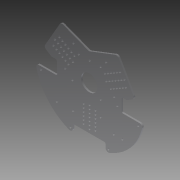
# Autodesk Inventor part: Motor Mount Plate
Saved by Autodesk Inventor 2015 (Build 190159000, 159)
## iProperties
Created: 2016-02-17
Part Number: Motor Mount Plate
Material: Polycarbonate, Clear
Document SubType Name: Modeling
Designer: 23902
Density: 1.2 g/cm^3
Appearance: Polycarbonate - Clear
Mass: 81.7977 g
Surface Area: 498.85 cm^2
Volume: 68.1648 cm^3
Author: 23902
Autodesk Inventor part; units mm, degrees
ref_plane "YZ Plane" through (0, 0, 0) normal (1, 0, 0) x (0, 1, 0)
ref_plane "XZ Plane" through (0, 0, 0) normal (0, 1, 0) x (-1, 0, 0)
ref_plane "XY Plane" through (0, 0, 0) normal (0, 0, 1) x (1, 0, 0)
sketch "Sketch1" plane through (0, 0, 0) normal (0, 1, 0) x (-1, 0, 0)
  circle A0 centre (63.7847, 36.7947) radius 1.65
  circle A1 centre (58.2854, 33.6197) radius 1.65
  circle A2 centre (52.7862, 30.4447) radius 1.65
  circle A3 centre (47.2869, 27.2697) radius 1.65
  circle A4 centre (41.7877, 24.0947) radius 1.65
  circle A5 centre (36.2884, 20.9197) radius 1.65
  circle A6 centre (30.7891, 17.7447) radius 1.65
  circle A7 centre (55.675, 44.6411) radius 1.65
  circle A8 centre (50.1758, 41.4661) radius 1.65
  circle A9 centre (44.6765, 38.2911) radius 1.65
  circle A10 centre (39.1772, 35.1161) radius 1.65
  circle A11 centre (33.678, 31.9411) radius 1.65
  circle A12 centre (28.1787, 28.7661) radius 1.65
  circle A13 centre (66.525, 25.8483) radius 1.65
  circle A14 centre (61.0258, 22.6733) radius 1.65
  circle A15 centre (55.5265, 19.4983) radius 1.65
  circle A16 centre (50.0272, 16.3233) radius 1.65
  circle A17 centre (44.528, 13.1483) radius 1.65
  circle A18 centre (39.0287, 9.9733) radius 1.65
  circle A19 centre (-63.6942, 36.7947) radius 1.65
  circle A20 centre (-58.195, 33.6197) radius 1.65
  circle A21 centre (-52.6957, 30.4447) radius 1.65
  circle A22 centre (-47.1965, 27.2697) radius 1.65
  circle A23 centre (-41.6972, 24.0947) radius 1.65
  circle A24 centre (-36.1979, 20.9197) radius 1.65
  circle A25 centre (-30.6987, 17.7447) radius 1.65
  circle A26 centre (-55.5846, 44.6411) radius 1.65
  circle A27 centre (-50.0853, 41.4661) radius 1.65
  circle A28 centre (-44.586, 38.2911) radius 1.65
  circle A29 centre (-39.0868, 35.1161) radius 1.65
  circle A30 centre (-33.5875, 31.9411) radius 1.65
  circle A31 centre (-28.0883, 28.7661) radius 1.65
  circle A32 centre (-66.4346, 25.8483) radius 1.65
  circle A33 centre (-60.9353, 22.6733) radius 1.65
  circle A34 centre (-55.436, 19.4983) radius 1.65
  circle A35 centre (-49.9368, 16.3233) radius 1.65
  circle A36 centre (-44.4375, 13.1483) radius 1.65
  circle A37 centre (-38.9383, 9.9733) radius 1.65
  circle A38 centre (0.0452, -73.6053) radius 1.65
  circle A39 centre (0.0452, -67.2553) radius 1.65
  circle A40 centre (0.0452, -60.9053) radius 1.65
  circle A41 centre (0.0452, -54.5553) radius 1.65
  circle A42 centre (0.0452, -48.2053) radius 1.65
  circle A43 centre (0.0452, -41.8553) radius 1.65
  circle A44 centre (0.0452, -35.5053) radius 1.65
  circle A45 centre (10.8952, -70.5053) radius 1.65
  circle A46 centre (10.8952, -64.1553) radius 1.65
  circle A47 centre (10.8952, -57.8053) radius 1.65
  circle A48 centre (10.8952, -51.4553) radius 1.65
  circle A49 centre (10.8952, -45.1053) radius 1.65
  circle A50 centre (10.8952, -38.7553) radius 1.65
  circle A51 centre (-10.8048, -70.5053) radius 1.65
  circle A52 centre (-10.8048, -64.1553) radius 1.65
  circle A53 centre (-10.8048, -57.8053) radius 1.65
  circle A54 centre (-10.8048, -51.4553) radius 1.65
  circle A55 centre (-10.8048, -45.1053) radius 1.65
  circle A56 centre (-10.8048, -38.7553) radius 1.65
  circle A57 centre (-29.9548, 47.4947) radius 1.6
  circle A58 centre (30.0452, 47.4947) radius 1.6
  circle A59 centre (35.0452, -88.3229) radius 1.6
  circle A60 centre (-34.9548, -88.3229) radius 1.6
  circle A61 centre (-89.3029, -23.9461) radius 1.6
  circle A62 centre (89.3934, -23.9461) radius 1.6
  circle A63 centre (-20.3391, -44.6576) radius 1.6079
  circle A64 centre (30.4218, -59.8922) radius 1.6079
  circle A65 centre (-44.4606, -59.8922) radius 1.6079
  circle A66 centre (-50.7872, -11.6704) radius 1.6079
  circle A67 centre (-20.3391, -16.7486) radius 1.6079
  circle A68 centre (31.6913, -11.6704) radius 1.6079
  circle A69 centre (0.0452, -0.0053) radius 15
  circle A70 centre (-19.9548, 34.9947) radius 1.6
  circle A71 centre (20.0452, 34.9947) radius 1.6
  circle A72 centre (60.1493, -60.1094) radius 1.6
  circle A73 centre (-60.0588, -60.1094) radius 1.6
  circle A74 centre (0.0452, 34.9947) radius 1.6
  circle A75 centre (45.0452, -0.0053) radius 1.6
  circle A76 centre (-44.9548, -0.0053) radius 1.6
  line L0 (0.0452, -80.0053) -> (-15.8048, -80.0053)
  line L1 (69.3273, 39.9947) -> (54.1439, 66.293)
  line L2 (-69.2368, 39.9947) -> (-54.0534, 66.293)
  line L3 (1.8413, 50.686) -> (48.0177, 68.4593)
  line L4 (-1.7508, 50.686) -> (-47.9273, 68.4593)
  arc A77 (-47.9273, 68.4593) -> (-54.0534, 66.293) centre (-49.7233, 63.793) ccw
  arc A78 (54.1439, 66.293) -> (48.0177, 68.4593) centre (49.8138, 63.793) ccw
  arc A79 (-1.7508, 50.686) -> (1.8413, 50.686) centre (0.0452, 55.3523) ccw
  line L5 (0.0452, -80.0053) -> (-27.9548, -80.0053)
  line L6 (-29.9548, -82.0053) -> (-29.9548, -88.3229)
  arc A80 (-44.5963, -89.4879) -> (-36.7969, -92.9712) centre (0.0452, -0.0053) ccw
  arc A81 (-36.7969, -92.9712) -> (-29.9548, -88.3229) centre (-34.9548, -88.3229) ccw
  arc A82 (-27.9548, -80.0053) -> (-29.9548, -82.0053) centre (-27.9548, -82.0053) ccw
  line L7 (0.0452, -80.0053) -> (15.8952, -80.0053)
  line L8 (0.0452, -80.0053) -> (28.0452, -80.0053)
  arc A83 (30.0452, -82.0053) -> (28.0452, -80.0053) centre (28.0452, -82.0053) ccw
  line L9 (30.0452, -82.0053) -> (30.0452, -88.3229)
  arc A84 (36.8873, -92.9712) -> (44.6868, -89.4879) centre (0.0452, -0.0053) ccw
  arc A85 (30.0452, -88.3229) -> (36.8873, -92.9712) centre (35.0452, -88.3229) ccw
  line L10 (-69.2368, 39.9947) -> (-80.8207, 19.9307)
  line L11 (-89.3029, -17.9461) -> (-92.1433, -17.9461)
  line L12 (-89.3029, -17.9461) -> (-71.3029, -17.9461)
  line L13 (-69.7888, 7.357) -> (-79.137, 13.1885)
  arc A86 (-96.9953, -24.1535) -> (-44.5963, -89.4879) centre (0.0452, -0.0053) ccw
  arc A87 (-92.1433, -17.9461) -> (-96.9953, -24.1535) centre (-92.1433, -22.9461) ccw
  arc A88 (-80.8207, 19.9307) -> (-79.137, 13.1885) centre (-76.4906, 17.4307) ccw
  line L14 (69.3273, 39.9947) -> (80.9112, 19.9307)
  arc A89 (79.2274, 13.1885) -> (80.9112, 19.9307) centre (76.5811, 17.4307) ccw
  arc A90 (44.6868, -89.4879) -> (97.0858, -24.1535) centre (0.0452, -0.0053) ccw
  arc A91 (97.0858, -24.1535) -> (92.2337, -17.9461) centre (92.2337, -22.9461) ccw
  line L15 (-71.3029, -17.9461) -> (-69.3029, -17.9461)
  line L16 (-69.3029, -17.9461) -> (-61.3029, -17.9461)
  line L17 (-59.3029, -15.9461) -> (-59.3029, 5.0539)
  line L18 (-61.3029, 7.0539) -> (-68.7302, 7.0539)
  arc A92 (-61.3029, -17.9461) -> (-59.3029, -15.9461) centre (-61.3029, -15.9461) ccw
  arc A93 (-59.3029, 5.0539) -> (-61.3029, 7.0539) centre (-61.3029, 5.0539) ccw
  arc A94 (-69.7888, 7.357) -> (-68.7302, 7.0539) centre (-68.7302, 9.0539) ccw
  line L19 (89.3934, -17.9461) -> (92.2337, -17.9461)
  line L20 (89.3934, -17.9461) -> (71.3934, -17.9461)
  line L21 (69.8792, 7.357) -> (79.2274, 13.1885)
  arc A95 (68.8207, 7.0539) -> (69.8792, 7.357) centre (68.8207, 9.0539) ccw
  line L22 (71.3934, -17.9461) -> (69.3934, -17.9461)
  line L23 (69.3934, -17.9461) -> (61.3934, -17.9461)
  line L24 (59.3934, -15.9461) -> (59.3934, 5.0539)
  arc A96 (61.3934, 7.0539) -> (59.3934, 5.0539) centre (61.3934, 5.0539) ccw
  arc A97 (59.3934, -15.9461) -> (61.3934, -17.9461) centre (61.3934, -15.9461) ccw
  line L25 (61.3934, 7.0539) -> (68.8207, 7.0539)
  constraints: 98 centre point, 52 end point, 42 point on circle, 2 point on line
extrude "Extrusion2" add sketch "Sketch1" along normal blind 3
body "Solid2"
